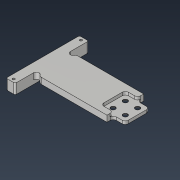
# Autodesk Inventor part: Kicker Chip
Saved by Autodesk Inventor 2022.1 (Build 261234020, 234B)
## iProperties
Part Number: Kicker Chip
Material: Aluminium 6061
Document SubType Name: Modeling
Designer: rYan
Mass: 16.7701 g
Surface Area: 40.2815 cm^2
Volume: 6.21115 cm^3
Density: 2.7 g/cm^3
Appearance: Aluminium - flach
Author: rYan
Autodesk Inventor part; units mm, degrees
ref_plane "YZ Plane" through (0, 0, 0) normal (1, 0, 0) x (0, 1, 0)
ref_plane "XZ Plane" through (0, 0, 0) normal (0, 1, 0) x (-1, 0, 0)
ref_plane "XY Plane" through (0, 0, 0) normal (0, 0, 1) x (1, 0, 0)
sketch "Skizze1" plane through (0, 0, 0) normal (0, 0, 1) x (1, 0, 0)
  line L0 (-6, 12) -> (48, 12)
  line L1 (48, 12) -> (48, -12)
  line L2 (48, -12) -> (-6, -12)
  line L3 (-16.8, 0) -> (58.8, 0) projected
  line L4 (0, 16.8) -> (0, -16.8) projected
  line L5 (-6, 12) -> (-6, -12)
  point P0 (0, 0)
  dimension "d2" = 24
  dimension "d3" = 54
  dimension "d59" = 6
  constraints: 8 end point, 1 horizontal, 1 parallel, 1 perpendicular, 1 point on line, 1 vertical, 1 other
  measures "d2" distance of L0.end L1.end
  measures "d3" distance of L0.start L0.end
  measures "d59" distance between parallel lines of L5 L4
extrude "Extrusion1" add sketch "Skizze1" along normal blind 6
sketch "Skizze2" plane through (0, 0, 0) normal (0, 0, -1) x (-1, 0, 0)
  line L0 (-48, -12) -> (6, -12) projected
  line L1 (-48, 12) -> (-48, -12) projected
  line L2 (-48, 12) -> (6, 12) projected
  line L3 (6, -12) -> (-48, -12)
  line L4 (-48, -12) -> (-48, 12)
  line L5 (-48, 12) -> (6, 12)
  line L6 (6, 12) -> (6, -12)
  point P0 (0, 0)
  constraints: 8 end point, 2 parallel, 1 horizontal, 1 perpendicular
extrude "Extrusion2" cut sketch "Skizze2" against normal blind 2
sketch "Skizze3" plane through (0, 0, 2) normal (0, 0, -1) x (-1, 0, 0)
  line L0 (6, -12) -> (-48, -12) projected
  line L1 (-48, -12) -> (-48, 12) projected
  line L2 (-48, 12) -> (6, 12) projected
  line L3 (-48, -12) -> (-44, -12)
  line L4 (-44, -12) -> (-44, 12)
  line L5 (-44, 12) -> (-48, 12)
  line L6 (-48, 12) -> (-48, -12)
  point P0 (0, 0)
  point P1 (0, -12.5)
  dimension "d9" = 4
  constraints: 8 end point, 2 parallel, 1 horizontal, 1 perpendicular, 1 point on line, 1 other
  measures "d9" distance between parallel lines of L1 L4
extrude "Extrusion3" [suppressed]
sketch "Skizze4" plane through (0, 0, 6) normal (0, 0, 1) x (1, 0, 0)
  line L0 (48, -12) -> (48, 12) projected
  line L1 (-17, 0) -> (60, 0) projected
  point P0 (0, 0)
  point P1 (46, 0)
  dimension "d12" = 2
  constraints: 1 point on line
  measures "d12" distance from line of L0 point (46, 0)
hole "Bohrung1" [suppressed]
pattern_linear "Rechteckige Anordnung1" [suppressed]
sketch "Skizze7" plane through (0, 0, 2) normal (0, 0, -1) x (-1, 0, 0)
  line L0 (6, -12) -> (-48, -12) projected
  line L1 (6, 12) -> (6, -12) projected
  line L2 (-48, 12) -> (6, 12) projected
  line L3 (-48, 12) -> (6, 12) projected
  line L4 (6, -12) -> (0, -12)
  line L5 (0, -12) -> (0, 12)
  line L6 (0, 12) -> (6, 12)
  line L7 (6, 12) -> (6, -12)
  line L8 (-48, -12) -> (-48, 12) projected
  point P0 (0, 0)
  point P1 (-44, 12)
  constraints: 8 end point, 2 parallel, 1 horizontal, 1 midpoint, 1 perpendicular, 1 point on line
extrude "Extrusion4" add sketch "Skizze7" along normal blind 2.8 contours L0 L5 L2 L1
sketch "Skizze8" plane through (0, 0, -0.8) normal (0, 0, -1) x (-1, 0, 0)
  line L0 (6, -12) -> (6, 12) projected
  line L1 (6, 12) -> (0, 12) projected
  line L2 (0, 12) -> (0, -12) projected
  line L3 (0, -12) -> (6, -12) projected
  line L4 (-58.8, 0) -> (16.8, 0) projected
  line L5 (6, 12) -> (0, 12)
  line L6 (0, 12) -> (0, 24)
  line L7 (0, 24) -> (6, 24)
  line L8 (6, 24) -> (6, 12)
  line L9 (6, -12) -> (-48, -12) projected
  line L10 (6, -12) -> (0, -12)
  line L11 (0, -12) -> (0, -24)
  line L12 (0, -24) -> (6, -24)
  line L13 (6, -24) -> (6, -12)
  line L14 (6, -12) -> (6, 12) projected
  dimension "d67" = 48
  constraints: 16 end point, 5 point on line, 4 parallel, 2 horizontal, 2 perpendicular, 1 collinear, 1 other
  measures "d67" distance between parallel lines of L12 L7
extrude "Extrusion5" add sketch "Skizze8" against normal up to surface (6.8 mm away)
sketch "Skizze9" plane through (0, 0, 6) normal (0, 0, 1) x (1, 0, 0)
  line L0 (0, -12) -> (48, -12) projected
  line L1 (48, -12) -> (48, 12) projected
  line L2 (48, 12) -> (0, 12) projected
  line L3 (0, 24) -> (0, 12) projected
  line L4 (-6, 24) -> (0, 24) projected
  line L5 (-6, -24) -> (-6, 24) projected
  line L6 (0, -24) -> (-6, -24) projected
  line L7 (0, -12) -> (0, -24) projected
  line L8 (48, 12) -> (0, 12) projected
  arc A0 (0, 12) -> (3.6, 12) centre (1.8, 12) ccw
  line L9 (0, -12) -> (48, -12) projected
  arc A1 (3.6, -12) -> (0, -12) centre (1.8, -12) ccw
  line L10 (-16.8, 0) -> (58.8, 0) projected
  point P0 (0, 0)
  point P1 (44, 12)
  point P2 (44, -12)
  dimension "d68" = 1.8
  constraints: 4 point on circle, 2 centre point, 2 point on line, 2 tangent, 1 other
  measures "d68" radius of A0
extrude "Extrusion6" cut sketch "Skizze9" against normal through all contours A1 L0 | A0 L2
fillet "Rundung1" radius 2 4 edges at (0, -12, 4) (3.6, -12, 4) (0, 12, 4) (3.6, 12, 4)
sketch "Skizze10" plane through (0, 0, -0.8) normal (0, 0, -1) x (-1, 0, 0)
  line L0 (0, -24) -> (0, 24) projected
  line L1 (-58.8, 0) -> (16.8, 0) projected
  line L2 (0, -22) -> (6, -22) construction
  line L3 (6, 24) -> (6, -24) projected
  point P0 (0, 0)
  point P1 (3, -22)
  point P2 (3, 22)
  dimension "d72" = 22
  constraints: 2 end point, 2 point on line, 1 midpoint, 1 symmetric about line
  measures "d72" distance between parallel lines of L1 L2
hole "Bohrung4" at (-3, -22, -0.8) at (-3, 22, -0.8) direction (0, 0, 1) diameter 1.567 end through all thread size "M2x0.4" class "6H" standard "ISO Metric profile"
fillet "Rundung2" radius 1 4 edges at (0, 24, 2.6) (-6, 24, 2.6) (0, -24, 2.6) (-6, -24, 2.6)
sketch "Skizze11" plane through (0, 0, -0.8) normal (0, 0, -1) x (-1, 0, 0)
  arc A0 (5, -24) -> (6, -23) centre (5, -23) ccw projected
  line L0 (6, 23) -> (6, -23) projected
  arc A1 (6, 23) -> (5, 24) centre (5, 23) ccw projected
  line L1 (1, 24) -> (5, 24) projected
  arc A2 (1, 24) -> (0, 23) centre (1, 23) ccw projected
  line L2 (0, -23) -> (0, 23) projected
  arc A3 (0, -23) -> (1, -24) centre (1, -23) ccw projected
  line L3 (5, -24) -> (1, -24) projected
  circle A4 centre (3, -22) radius 0.7835 projected
  circle A5 centre (3, 22) radius 0.7835 projected
  point P0 (0, 0)
extrude "Extrusion7" cut sketch "Skizze11" against normal blind 0.2
sketch "Skizze12" plane through (0, 0, 6) normal (0, 0, 1) x (1, 0, 0)
  line L0 (48, -12) -> (48, 12) construction
  line L1 (-16.8, 0) -> (58.8, 0) construction
  line L2 (48, -12) -> (48, 12) projected
  line L3 (48, 8) -> (42, 8)
  line L4 (40, 6) -> (40, -6)
  line L5 (42, -8) -> (48, -8)
  line L6 (48, -8) -> (48, 8)
  arc A0 (42, 8) -> (40, 6) centre (42, 6) ccw
  arc A1 (40, -6) -> (42, -8) centre (42, -6) ccw
  point P0 (0, 0)
  dimension "d83" = 2
  dimension "d84" = 4
  dimension "d85" = 8
  constraints: 8 end point, 4 point on circle, 4 tangent, 2 centre point, 2 parallel, 1 equal radius, 1 horizontal, 1 perpendicular, 1 point on line, 2 other
  measures "d83" radius of A0
  measures "d84" distance from line of L0.end L3
  measures "d85" distance between parallel lines of L0 L4
extrude "Extrusion8" cut sketch "Skizze12" against normal blind 2
sketch "Skizze13" plane through (0, 0, 2) normal (0, 0, -1) x (-1, 0, 0)
  line L0 (-48, -12) -> (-48, 12) construction
  line L1 (-58.8, 0) -> (16.8, 0) construction
  line L2 (-48, -7.9) -> (-53.8, -7.9)
  line L3 (-55.8, -5.9) -> (-55.8, 5.9)
  line L4 (-53.8, 7.9) -> (-48, 7.9)
  line L5 (-48, 7.9) -> (-48, -7.9)
  arc A0 (-55.8, -5.9) -> (-53.8, -7.9) centre (-53.8, -5.9) ccw
  arc A1 (-53.8, 7.9) -> (-55.8, 5.9) centre (-53.8, 5.9) ccw
  point P0 (0, 0)
  dimension "d88" = 2
  dimension "d89" = 4.1
  dimension "d90" = 7.8
  constraints: 8 end point, 4 point on circle, 4 tangent, 2 centre point, 2 parallel, 1 equal radius, 1 horizontal, 1 perpendicular, 1 point on line, 2 other
  measures "d88" radius of A0
  measures "d89" distance from line of L0.start L2
  measures "d90" distance between parallel lines of L3 L0
extrude "Extrusion9" add sketch "Skizze13" against normal blind 2
sketch "Skizze14" plane through (0, 0, 2) normal (0, 0, -1) x (-1, 0, 0)
  line L0 (-48, -12) -> (-48, -7.9) construction
  line L1 (-68.16, 0) -> (18.36, 0) construction
  line L2 (-44, -4) -> (-52, -4) construction
  line L3 (-52, -4) -> (-52, 4) construction
  line L4 (-52, 4) -> (-44, 4) construction
  line L5 (-44, 4) -> (-44, -4) construction
  point P0 (0, 0)
  dimension "d93" = 8
  dimension "d94" = 8
  constraints: 8 end point, 4 coincident, 2 parallel, 1 horizontal, 1 perpendicular, 2 other
  measures "d93" distance of L2.start L2.end
  measures "d94" distance of L4.end L2.start
hole "Bohrung5" at (44, -4, 2) at (52, -4, 2) at (52, 4, 2) at (44, 4, 2) direction (0, 0, 1) diameter 3 end through all countersink diameter 6.7 countersink angle 90
fillet "Rundung3" radius 2 4 edges at (48, -8, 5) (48, -7.9, 3) (48, 8, 5) (48, 7.9, 3)
